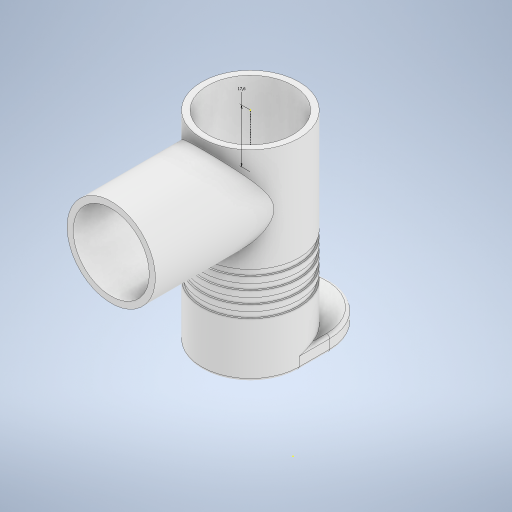
# Autodesk Inventor part: wieszak
Saved by Autodesk Inventor 2024 (Build 280153000, 153)
## iProperties
Created: 2024-06-07
Part Number: wieszak
Material: PC/ABS Plastic
Document SubType Name: Modeling
Designer: Miki
Density: 1.1 g/cm^3
Appearance: Smooth - White
Author: Miki
Autodesk Inventor part; units mm, degrees
ref_plane "YZ Plane" through (0, 0, 0) normal (1, 0, 0) x (0, 1, 0)
ref_plane "XZ Plane" through (0, 0, 0) normal (0, 1, 0) x (-1, 0, 0)
ref_plane "XY Plane" through (0, 0, 0) normal (0, 0, 1) x (1, 0, 0)
sketch "Sketch3" plane through (0, 0, 0) normal (0, 1, 0) x (-1, 0, 0)
  arc A0 (23.3543, -35.423) -> (55.3543, -35.423) centre (39.3543, -35.423) ccw
  arc A1 (55.3543, -25.423) -> (23.3543, -25.423) centre (39.3543, -25.423) ccw
  line L0 (39.3543, -25.423) -> (39.3543, -35.423) construction
  line L1 (39.3543, -25.423) -> (55.3543, -25.423) construction
  line L2 (39.3543, -35.423) -> (55.3543, -35.423) construction
  line L3 (39.3543, -25.423) -> (23.3543, -25.423) construction
  line L4 (39.3543, -35.423) -> (23.3543, -35.423) construction
  line L5 (23.3543, -25.423) -> (23.3543, -35.423)
  line L6 (55.3543, -25.423) -> (55.3543, -35.423)
  point P0 (0, 0)
  dimension "d7" = 32
  dimension "d8" = 32
  dimension "d9" = 10
  constraints: 14 end point, 4 horizontal, 4 point on circle, 2 centre point, 2 tangent, 2 vertical
  measures "d7" diameter of A0
  measures "d8" diameter of A1
  measures "d9" distance of L0.start L0.end
extrude "Extrusion2" add sketch "Sketch3" along normal blind 5
sketch "Sketch4" plane through (0, 5, 0) normal (0, 1, 0) x (1, 0, 0)
  arc A0 (-55.3543, 25.423) -> (-23.3543, 25.423) centre (-39.3543, 25.423) ccw projected
  line L0 (-55.3543, 25.423) -> (-39.3543, 25.423) construction
  circle A1 centre (-39.3543, 25.423) radius 16
  circle A2 centre (-39.3543, 25.423) radius 14
  point P0 (0, 0)
  point P1 (-23.3543, 25.423)
  dimension "d12" = 16
  dimension "d13" = 32
  dimension "d14" = 28
  constraints: 2 centre point, 2 coincident, 2 end point, 1 horizontal
  measures "d12" distance of L0.start L0.end
  measures "d13" diameter of A1
  measures "d14" diameter of A2
extrude "Extrusion3" add sketch "Sketch4" along normal blind 13
sketch "Sketch5" plane through (-39.3543, 18, -25.423) normal (0, 1, 0) x (1, 0, 0)
  circle A0 centre (0, 0) radius 15.5
  circle A1 centre (0, 0) radius 14
  point P0 (39.3543, -25.423)
  dimension "d17" = 31
  constraints: 2 centre point, 1 coincident
  measures "d17" diameter of A0
extrude "Extrusion4" add sketch "Sketch5" along normal blind 2
sketch "Sketch6" plane through (-39.3543, 20, -25.423) normal (0, 1, 0) x (1, 0, 0)
  circle A0 centre (0, 0) radius 14
  circle A1 centre (0, 0) radius 16
  point P0 (39.3543, -25.423)
  constraints: 2 centre point, 1 coincident
extrude "Extrusion5" add sketch "Sketch6" along normal blind 2
sketch "Sketch7" plane through (-39.3543, 22, -25.423) normal (0, 1, 0) x (1, 0, 0)
  circle A0 centre (0, 0) radius 14
  circle A1 centre (0, 0) radius 15.5
  point P0 (39.3543, -25.423)
  dimension "d22" = 31
  constraints: 2 centre point, 1 coincident
  measures "d22" diameter of A1
extrude "Extrusion6" add sketch "Sketch7" along normal blind 2
sketch "Sketch8" plane through (-39.3543, 24, -25.423) normal (0, 1, 0) x (1, 0, 0)
  circle A0 centre (0, 0) radius 14
  arc A1 (-16, 0) -> (16, 0) centre (0, 0) ccw projected
  circle A2 centre (0, 0) radius 16
  point P0 (39.3543, -25.423)
  point P1 (16, 0)
  constraints: 1 centre point, 1 coincident, 3 other
extrude "Extrusion7" add sketch "Sketch8" along normal blind 2
sketch "Sketch10" plane through (-39.3543, 26, -25.423) normal (0, 1, 0) x (1, 0, 0)
  circle A0 centre (0, 0) radius 14
  circle A1 centre (0, 0) radius 15.5
  point P0 (39.3543, -25.423)
  dimension "d27" = 31
  constraints: 2 centre point, 1 coincident
  measures "d27" diameter of A1
extrude "Extrusion8" add sketch "Sketch10" along normal blind 2
sketch "Sketch11" plane through (-39.3543, 28, -25.423) normal (0, 1, 0) x (1, 0, 0)
  circle A0 centre (0, 0) radius 14
  circle A1 centre (0, 0) radius 16
  point P0 (39.3543, -25.423)
  constraints: 2 centre point, 1 coincident
extrude "Extrusion9" add sketch "Sketch11" along normal blind 2
sketch "Sketch12" plane through (-39.3543, 30, -25.423) normal (0, 1, 0) x (1, 0, 0)
  circle A0 centre (0, 0) radius 14
  circle A1 centre (0, 0) radius 15.5
  point P0 (39.3543, -25.423)
  dimension "d32" = 31
  constraints: 2 centre point, 1 coincident
  measures "d32" diameter of A1
extrude "Extrusion10" add sketch "Sketch12" along normal blind 2
sketch "Sketch13" plane through (-39.3543, 32, -25.423) normal (0, 1, 0) x (1, 0, 0)
  circle A0 centre (0, 0) radius 14
  circle A1 centre (0, 0) radius 16
  point P0 (39.3543, -25.423)
  constraints: 2 centre point, 1 coincident
extrude "Extrusion11" add sketch "Sketch13" along normal blind 34
sketch3d "3D Sketch1"
sketch "Sketch14" plane through (0, 0, 0) normal (0, 0, 1) x (1, 0, 0)
  point P0 (0, 0)
sketch "Sketch15" plane through (0, 0, 0) normal (0, 0, 1) x (1, 0, 0)
  line L0 (-53.3543, 66) -> (-25.3543, 66) construction
  line L1 (-39.3543, 66) -> (-39.3543, 48.4) construction
  circle A0 centre (-39.3543, 48.4) radius 14.5
  point P0 (0, 0)
  dimension "d38" = 17.6
  dimension "d39" = 29
  constraints: 2 end point, 1 centre point, 1 coincident, 1 midpoint, 1 vertical
  measures "d38" distance of L1.start L1.end
  measures "d39" diameter of A0
sketch "Sketch16" plane through (0, 0, 0) normal (0, 0, 1) x (1, 0, 0)
  circle A0 centre (-39.3544, 48.4) radius 13.5
  point P0 (0, 0)
  dimension "d40" = 27
  constraints: 1 centre point
  measures "d40" diameter of A0
extrude "Extrusion13" cut sketch "Sketch16" against normal up to surface round surface about axis through (-39.3543, 32, -25.423) along (0, 1, 0) radius 16 far side no
extrude "Extrusion14" add sketch "Sketch15" against normal up to surface round surface about axis through (-39.3543, 32, -25.423) along (0, 1, 0) radius 16 far side no
sketch "Sketch19" plane through (-39.3543, 48.4, 0) normal (0, 0, 1) x (1, 0, 0)
  circle A0 centre (0, 0) radius 14.5
  point P0 (39.3543, -48.4)
  constraints: 1 centre point
extrude "Extrusion15" add sketch "Sketch19" along normal blind 20.25
sketch "Sketch20" plane through (-39.3543, 48.4, 20.25) normal (0, 0, 1) x (1, 0, 0)
  circle A0 centre (0, 0) radius 12.5
  point P0 (39.3543, -48.4)
  dimension "d53" = 25
  constraints: 1 centre point
  measures "d53" diameter of A0
extrude "Extrusion16" cut sketch "Sketch20" against normal up to surface round surface about axis through (-39.3543, 32, -25.423) along (0, 1, 0) radius 16 far side no
fillet "Fillet1" radius 1 7 edges at (-39.3543, 0, -51.423) (-55.3543, 0, -30.423) (-39.3543, 0, -9.423) (-23.3543, 0, -30.423) (-39.3543, 5, -51.423) (-55.3543, 5, -30.423) (-23.3543, 5, -30.423)
body "Solid2"
